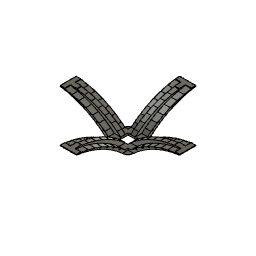
bear_overhang_big_50-80 (Autodesk Fusion 360 design; units mm, degrees)
Autodesk Fusion 360 part; units mm, degrees
sketch "arm" plane through (0, 0, 0) normal (0, 1, 0) x (1, 0, 0) in component "bear_overhang_big_50-80"
  line L0 (15, 0) -> (10, 0)
  line L1 (27.7666, -9.8) -> (34.6948, -13.8)
  line L2 (15, 0) -> (21.1971, -5.2)
  line L3 (21.1971, -5.2) -> (27.7666, -9.8)
  line L4 (0, -2) -> (0, 0)
  line L5 (0, 0) -> (0, -27.1786) construction
  line L6 (29.6948, -13.8) -> (22.7666, -9.8)
  line L7 (34.6948, -13.8) -> (29.6948, -13.8) construction
  line L8 (27.7666, -9.8) -> (22.7666, -9.8) construction
  line L9 (21.1971, -5.2) -> (16.1971, -5.2) construction
  line L10 (22.7666, -9.8) -> (16.1971, -5.2)
  line L11 (16.1971, -5.2) -> (10, 0)
  line L12 (34.6948, -13.8) -> (41.9861, -17.2)
  line L13 (41.9861, -17.2) -> (49.6791, -20)
  line L14 (29.6948, -13.8) -> (36.9861, -17.2)
  line L15 (36.9861, -17.2) -> (44.6791, -20)
  line L16 (41.9861, -17.2) -> (36.9861, -17.2) construction
  line L17 (10, 0) -> (0, 0)
  line L18 (0, -2) -> (12.3835, -2)
  line L19 (5.3835, -2) -> (9.1971, -5.2)
  line L20 (9.1971, -5.2) -> (15.7666, -9.8)
  line L21 (15.7666, -9.8) -> (22.6948, -13.8)
  line L22 (22.6948, -13.8) -> (29.9861, -17.2)
  line L23 (29.9861, -17.2) -> (37.6791, -20)
  line L24 (49.6791, -20) -> (57.1432, -22)
  line L25 (57.1432, -22) -> (52.1432, -22) construction
  line L26 (45.1432, -22) -> (37.6791, -20)
  line L27 (44.6791, -20) -> (49.6791, -20) construction
  line L28 (44.6791, -20) -> (52.1432, -22)
  line L29 (45.1432, -22) -> (53.083, -23.4)
  line L30 (60.083, -23.4) -> (65.083, -23.4)
  line L31 (65.083, -23.4) -> (57.1432, -22)
  line L32 (52.1432, -22) -> (60.083, -23.4)
  line L33 (53.083, -23.4) -> (60.083, -23.4)
  line L34 (53.083, -23.4) -> (53.083, -24)
  line L35 (53.083, -24) -> (65.083, -24)
  line L36 (65.083, -24) -> (65.083, -23.4)
  line L37 (60.083, -23.4) -> (60.083, -24)
  dimension "d9" = 5.2
  dimension "d10" = 4.6
  dimension "d13" = 4
  dimension "d24" = 50
  dimension "d25" = 55
  dimension "d26" = 60
  dimension "d45" = 7.6
  dimension "d46" = 7.6019
  dimension "d50" = 65
  dimension "d51" = 70
  dimension "d52" = 3.4
  dimension "d53" = 2.8
  dimension "d54" = 6.6254
  dimension "d55" = 7.0171
  dimension "d78" = 5
  dimension "d79" = 10
  dimension "d84" = 2
  dimension "d85" = 5.9118
  dimension "d98" = 7
  dimension "d99" = 75
  dimension "d100" = 10.1153
  dimension "d101" = 2
  dimension "d103" = 80
  dimension "d104" = 1.4
  dimension "d105" = 5.7588
  dimension "d108" = 0.6
  constraint horizontal L7
  constraint horizontal L8
  constraint horizontal L9
  constraint horizontal L0
  constraint coincident L4.end L5.start
  constraint horizontal L16
  constraint perpendicular L5 L17
  constraint parallel L0 L17
  constraint equal L0 L9
  constraint perpendicular L4 L17
  constraint coincident L11 L18.end
  constraint perpendicular L5 L18
  constraint coincident L18 L19.start
  constraint parallel L11 L19
  constraint parallel L10 L20
  constraint parallel L6 L21
  constraint parallel L14 L22
  constraint coincident L9 L19.end
  constraint coincident L7 L21.end
  constraint coincident L8 L20.end
  constraint parallel L15 L23
  constraint coincident L16 L22.end
  constraint horizontal L27
  constraint coincident L23.end L27
  constraint horizontal L25
  constraint parallel L26 L28
  constraint equal L8 L9
  constraint equal L7 L8
  constraint equal L7 L16
  constraint equal L16 L27
  constraint equal L25 L27
  constraint coincident L25 L26.start
  constraint horizontal L30
  constraint parallel L30 L33
  constraint parallel L29 L32
  constraint equal L25 L30
  constraint perpendicular L33 L34
  constraint perpendicular L34 L35
  constraint perpendicular L35 L36
  constraint coincident L35 L37.end
  constraint perpendicular L35 L37
  measures "d9" vertical distance of L2.end L0.start
  measures "d10" vertical distance of L2.end L1.start
  measures "d13" vertical distance of L1.end L1.start
  measures "d24" angle of L2 L5
  measures "d25" angle of L3 L5
  measures "d26" angle of L1 L5
  measures "d50" angle of L5 L12
  measures "d51" angle of L5 L13
  measures "d52" vertical distance of L1.end L12.end
  measures "d53" vertical distance of L13.end L12.end
  measures "d78" distance of L0.start L0.end
  measures "d79" distance of L4.end L0.end
  measures "d84" distance of L4.end L4.start
  measures "d98" distance of L18.end L19.start
  measures "d99" angle of L5 L24
  measures "d101" vertical distance of L13.end L24.end
  measures "d103" angle of L5 L31
  measures "d104" vertical distance of L24.end L30.end
  measures "d108" distance of L30.end L35.end
extrude "Extrude1" add sketch "arm" along normal mid plane 18 contours L0 L1 L2 L3 L6 L10 L11 L12 L13 L14 L15 L24 L28 L30 L31 L32 | L4 L11 L17 L18 | L30 L35 L36 L37 makes body 1 in component "bear_overhang_big_50-80"
extrude "Extrude2" add sketch "arm" along normal mid plane 5 contours L6 L10 L11 L14 L15 L18 L19 L20 L21 L22 L23 L26 L28 L29 L32 L33 | L33 L34 L35 L37 bodies 1 in component "bear_overhang_big_50-80"
sketch "angle_indication" plane through (0, -9, 0) normal (0, -1, 0) x (1, 0, 0) in component "bear_overhang_big_50-80"
  line L0 (21.1971, 5.2) -> (16.1971, 5.2)
  line L1 (27.7666, 9.8) -> (22.7666, 9.8)
  line L2 (34.6948, 13.8) -> (29.6948, 13.8)
  line L3 (41.9861, 17.2) -> (36.9861, 17.2)
  line L4 (18.6971, 5.2) -> (18.9827, 5.4)
  line L5 (18.9827, 5.4) -> (16.4827, 5.4)
  line L6 (25.2666, 9.8) -> (25.613, 10)
  line L7 (25.613, 10) -> (23.113, 10)
  line L8 (32.1948, 13.8) -> (32.6237, 14)
  line L9 (32.6237, 14) -> (30.1237, 14)
  line L10 (39.4861, 17.2) -> (40.0356, 17.4)
  line L11 (40.0356, 17.4) -> (37.5356, 17.4)
  line L12 (22.7666, 9.8) -> (16.1971, 5.2)
  line L13 (29.6948, 13.8) -> (22.7666, 9.8)
  line L14 (36.9861, 17.2) -> (29.6948, 13.8)
  line L15 (44.6791, 20) -> (36.9861, 17.2)
  line L16 (52.1432, 22) -> (44.6791, 20)
  line L17 (49.6791, 20) -> (44.6791, 20)
  line L18 (45.4255, 20.2) -> (47.9255, 20.2)
  line L19 (47.9255, 20.2) -> (47.1791, 20)
  line L20 (52.1432, 22) -> (57.1432, 22)
  line L21 (60.083, 23.4) -> (52.1432, 22)
  line L22 (54.6432, 22) -> (55.7774, 22.2)
  line L23 (55.7774, 22.2) -> (53.2774, 22.2)
  line L24 (60.083, 23.4) -> (65.083, 23.4)
  line L25 (60.083, 24) -> (60.083, 23.4)
  line L26 (65.083, 24) -> (60.083, 24)
  line L27 (65.083, 23.4) -> (65.083, 24)
  point P0 (21.1971, 5.2)
  point P1 (27.7666, 9.8)
  point P2 (34.6948, 13.8)
  point P3 (41.9861, 17.2)
  point P4 (49.6791, 20)
  point P5 (57.1432, 22)
  point P6 (65.083, 23.4)
  dimension "d68" = 0.2
  dimension "d69" = 0.2
  dimension "d70" = 0.2
  dimension "d71" = 0.2
  dimension "d102" = 0.2
  dimension "d109" = 0.2
  constraint midpoint L0 L4.start
  constraint midpoint L1 L6.start
  constraint midpoint L2 L8.start
  constraint midpoint L3 L10.start
  constraint parallel L0 L5
  constraint parallel L1 L7
  constraint parallel L2 L9
  constraint parallel L3 L11
  constraint coincident L11.end L15
  constraint coincident L3.end L14.start
  constraint coincident L2.end L13.start
  constraint coincident L1.end L12.start
  constraint coincident L0.end L12.end
  constraint parallel L4 L12
  constraint parallel L6 L13
  constraint parallel L8 L14
  constraint parallel L10 L15
  constraint coincident L9.end L14
  constraint coincident L7.end L13
  constraint coincident L5.end L12
  constraint coincident P0 L0.start
  constraint coincident P1 L1.start
  constraint coincident P2 L2.start
  constraint coincident P3 L3.start
  constraint coincident P4 L17.start
  constraint coincident L15.start L16.end
  constraint coincident L16 L18.start
  constraint parallel L17 L18
  constraint midpoint L17 L19.end
  constraint parallel L16 L19
  constraint coincident L16.start L20.start
  constraint coincident P5 L20.end
  constraint midpoint L20 L22.start
  constraint parallel L21 L22
  constraint coincident L21 L23.end
  constraint parallel L20 L23
  constraint coincident L21.start L24.start
  constraint horizontal L24
  constraint coincident P6 L24.end
  measures "d68" distance of L0 L5
  measures "d69" distance of L1 L7
  measures "d70" distance of L2 L9
  measures "d71" distance of L3 L11
  measures "d102" distance of L17 L18
  measures "d109" distance of L20 L23
extrude "Extrude2'" cut sketch "angle_indication" against normal blind 0.3 bodies 1 in component "bear_overhang_big_50-80"
mirror "Mirror1" about plane through (0, 0, 0) normal (0, 1, 0) of "Extrude2'" in component "bear_overhang_big_50-80"
pattern_circular "C-Pattern1" count 4 over 360 about axis through (0, 0, 1.75) along (0, 0, 1) of bodies 1 makes body 2 at (-2.5, 18.2434, 8.2667) makes body 3 at (-18.2434, -2.5, 8.2667) makes body 4 at (3, -5, 0) in component "bear_overhang_big_50-80"
combine "Combine1" operation add target body 1 tool bodies 4 3 2 in component "bear_overhang_big_50-80"
sketch "orientation_mark" plane through (0, 0, 0) normal (0, 0, -1) x (1, 0, 0) in component "bear_overhang_big_50-80"
  line L0 (-9, 9) -> (-15, 9)
  line L1 (9, -9) -> (15, -9)
  line L2 (-9, -9) -> (-9, -15)
  line L3 (9, -15) -> (9, -9)
  line L4 (15, 9) -> (9, 9)
  line L5 (9, 9) -> (9, 15)
  line L6 (-9, 15) -> (-9, 9)
  arc A0 (9, -15) -> (15, -9) centre (9, -9) ccw
  arc A1 (15, 9) -> (9, 15) centre (9, 9) ccw
  arc A2 (-9, 15) -> (-15, 9) centre (-9, 9) ccw
  arc A3 (-15, -9) -> (-9, -15) centre (-9, -9) ccw
  line L7 (-15, 9) -> (-15, -9)
  line L8 (-9, -15) -> (9, -15)
  line L9 (15, -9) -> (15, 9)
  line L10 (9, 15) -> (-9, 15)
  line L11 (-15, -9) -> (-9, -9)
  line L12 (0, 15) -> (0, -15) construction
  line L13 (-15, 0) -> (15, 0) construction
  line L14 (-5.3835, -2.5) -> (-5.3835, 2.5)
  line L15 (-2.5, 5.3835) -> (2.5, 5.3835)
  line L16 (5.3835, 2.5) -> (5.3835, -2.5)
  line L17 (2.5, -5.3835) -> (-2.5, -5.3835)
  line L18 (-5.3835, -2.5) -> (-5.3835, -5.3835)
  line L19 (-5.3835, -5.3835) -> (-2.5, -5.3835)
  line L20 (2.5, -5.3835) -> (5.3835, -5.3835)
  line L21 (5.3835, -5.3835) -> (5.3835, -2.5)
  line L22 (2.5, 5.3835) -> (5.3835, 5.3835)
  line L23 (5.3835, 5.3835) -> (5.3835, 2.5)
  arc A4 (-2.5, 5.3835) -> (-5.3835, 2.5) centre (-2.5, 2.5) ccw
  constraint coincident L2.end A3.end
  constraint coincident A3.start L7.end
  constraint coincident L0.end A2.end
  constraint coincident L6.start A2.start
  constraint coincident L5.end A1.end
  constraint coincident L1.end A0.end
  constraint coincident L3.start A0.start
  constraint tangent A0 L8
  constraint tangent A3 L8
  constraint tangent A2 L7
  constraint tangent A1 L10
  constraint coincident L4.start A1.start
  constraint midpoint L10 L12.start
  constraint midpoint L8 L12.end
  constraint midpoint L7 L13.start
  constraint midpoint L9 L13.end
  constraint coincident L14.start L18.start
  constraint parallel L14 L18
  constraint coincident L17.end L19.end
  constraint coincident L17.start L20.start
  constraint parallel L17 L20
  constraint coincident L16.end L21.end
  constraint parallel L16 L21
  constraint parallel L17 L19
  constraint coincident L15.end L22.start
  constraint parallel L15 L22
  constraint coincident L16.start L23.end
  constraint parallel L16 L23
  constraint tangent L15 A4
  constraint tangent L14 A4
  constraint coincident L15.start A4.start
  constraint coincident L14.end A4.end
extrude "Extrude3" add sketch "orientation_mark" against normal blind 0.2 contours L0 L6 A2 | L2 A3 L11 | L4 L5 A1 | L1 L3 A0 bodies 1 in component "bear_overhang_big_50-80"
extrude "Extrude4" cut sketch "orientation_mark" along normal up to surface (2 mm away) from surface at -2 contours L14 L15 L16 L17 L18 L19 L20 L21 L22 L23 A4 bodies 1 in component "bear_overhang_big_50-80"
component "bear_overhang_big_50-80" placed x (1, 0, 0) y (0, 1, 0) z (0, 0, 1) at (0, 0, 0)
equation "d9 = layer_height * 26"
equation "d10 = layer_height * 23"
equation "d13 = layer_height * 20"
equation "d31 = arm_width"
equation "layer_height = 0.2 mm"
equation "arm_width = 18 mm"
equation "arm_support_width = arm_width / 3"
equation "d52 = layer_height * 17"
equation "d53 = layer_height * 14"
equation "arm_layer_length = e_width + ( num_perimeters * 2 - 1 ) * e_spacing"
equation "d68 = layer_height"
equation "d69 = layer_height"
equation "d70 = layer_height"
equation "d71 = layer_height"
equation "d75 = -layer_height"
equation "e_width = 0.45 mm"
equation "e_spacing = 0.4071 mm"
equation "num_perimeters = 2"
equation "d101 = layer_height * 10"
equation "d102 = layer_height"
equation "d104 = layer_height * 7"
equation "num_bottom_layers = 4"
equation "num_top_layers = 3"
equation "d108 = num_top_layers * layer_height"
equation "d109 = layer_height"
